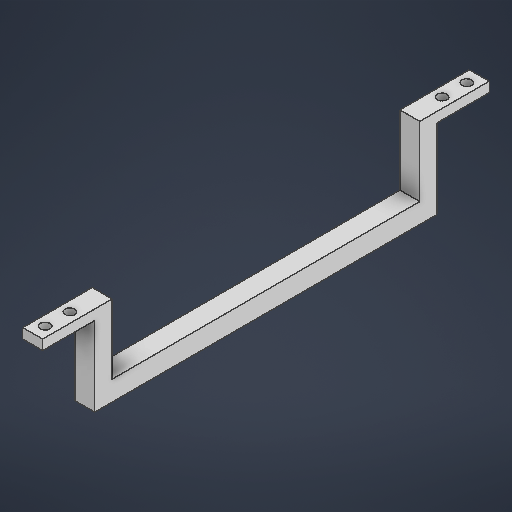
# Autodesk Inventor part: side_wall2
Saved by Autodesk Inventor 2026.1 (Build 301233000, 233)
## iProperties
Created: 2026-03-22
Part Number: side_wall2
Material: Generic
Document SubType Name: Modeling
Designer: emanuel
Density: 1 g/cm^3
Appearance: Default
Author: emanuel
Autodesk Inventor part; units mm, degrees
ref_plane "YZ Plane" through (0, 0, 0) normal (1, 0, 0) x (0, 1, 0)
ref_plane "XZ Plane" through (0, 0, 0) normal (0, 1, 0) x (-1, 0, 0)
ref_plane "XY Plane" through (0, 0, 0) normal (0, 0, 1) x (1, 0, 0)
sketch "Sketch1" plane through (0, 0, 0) normal (0, 1, 0) x (-1, 0, 0)
  circle A0 centre (0, 0) radius 2
  line L0 (0, 0) -> (0, -10)
  circle A1 centre (0, -10) radius 2
  line L1 (0, 0) -> (4, 0)
  line L2 (4, 0) -> (4, 5)
  line L3 (4, 5) -> (0, 5)
  line L4 (0, 5) -> (0, 0)
  line L5 (0, -10) -> (-4, -10)
  line L6 (-4, -10) -> (-4, -15)
  line L7 (-4, -15) -> (0, -15)
  line L8 (0, -15) -> (0, -10)
  line L9 (4, 5) -> (-4, 5)
  line L10 (-4, 5) -> (-4, -15)
  line L11 (-4, -15) -> (4, -15)
  line L12 (4, -15) -> (4, 5)
  line L13 (4, -15) -> (-4, -15)
  line L14 (-4, -15) -> (-4, -23)
  line L15 (-4, -23) -> (4, -23)
  line L16 (4, -23) -> (4, -15)
  line L17 (0, -10) -> (0, -85)
  line L18 (0, -85) -> (10, -85)
  circle A2 centre (0, -170) radius 2
  line L19 (0, -170) -> (0, -160)
  circle A3 centre (0, -160) radius 2
  line L20 (0, -170) -> (4, -170)
  line L21 (4, -170) -> (4, -175)
  line L22 (4, -175) -> (0, -175)
  line L23 (0, -175) -> (0, -170)
  line L24 (0, -160) -> (-4, -160)
  line L25 (-4, -160) -> (-4, -155)
  line L26 (-4, -155) -> (0, -155)
  line L27 (0, -155) -> (0, -160)
  line L28 (4, -175) -> (-4, -175)
  line L29 (-4, -175) -> (-4, -155)
  line L30 (-4, -155) -> (4, -155)
  line L31 (4, -155) -> (4, -175)
  line L32 (4, -155) -> (-4, -155)
  line L33 (-4, -155) -> (-4, -147)
  line L34 (-4, -147) -> (4, -147)
  line L35 (4, -147) -> (4, -155)
  dimension "d0" = 4
  dimension "d1" = 10
  dimension "d2" = 4
  dimension "d3" = 4
  dimension "d4" = 5
  dimension "d5" = 4
  dimension "d6" = 5
  dimension "d7" = 8
  dimension "d8" = 75
  dimension "d9" = 10
  constraints: 72 end point, 15 symmetric about line, 8 parallel, 5 perpendicular, 4 centre point, 4 coincident, 4 horizontal, 3 point on line, 1 vertical, 2 other
  measures "d0" diameter of A0
  measures "d1" distance of L0.start L0.end
  measures "d2" diameter of A1
  measures "d3" distance of L3.end L2.end
  measures "d4" distance of L2.end L1.end
  measures "d5" distance of L7.end L6.end
  measures "d6" distance of L6.end L5.end
  measures "d7" distance of L14.end L13.end
  measures "d8" distance of L5.start L17.end
  measures "d9" distance of L17.end L18.end
extrude "Extrusion1" add sketch "Sketch1" along normal blind 4 contours L1 L12 L11 L8 A1 L0 A0 | A0 L4 L3 L2 L1 | A0 L0 A1 L5 L10 L9 L4 | L16 L15 L17 L11 | A1 L8 L7 L6 L5 | L17 L15 L14 L7 | L20 L21 L22 L23 A2 | A2 L19 A3 L27 L30 L31 L20 | A2 L23 L28 L29 L24 A3 L19 | L30 L26 L33 L34 L35 | L24 L25 L26 L27 A3
sketch "Sketch2" plane through (0, 0, 0) normal (0, -1, 0) x (1, 0, 0)
  line L0 (4, -23) -> (-4, -23) projected
  line L1 (4, 5) -> (4, -23) projected
  line L2 (-4, -23) -> (4, -23)
  line L3 (4, -23) -> (4, -16)
  line L4 (4, -16) -> (-4, -16)
  line L5 (-4, -16) -> (-4, -23)
  line L6 (-4, -147) -> (4, -147) projected
  line L7 (-4, -147) -> (4, -147)
  line L8 (4, -147) -> (4, -154)
  line L9 (4, -154) -> (-4, -154)
  line L10 (-4, -154) -> (-4, -147)
  point P0 (0, 0)
  dimension "d12" = 7
  dimension "d13" = 7
  constraints: 16 end point, 4 parallel, 2 horizontal, 2 perpendicular, 2 point on line
  measures "d12" distance of L3.end L2.end
  measures "d13" distance of L7.end L8.end
extrude "Extrusion2" add sketch "Sketch2" along normal blind 32
sketch "Sketch3" plane through (0, -32, 0) normal (0, -1, 0) x (1, 0, 0)
  line L0 (4, -154) -> (4, -147) projected
  line L1 (-4, -16) -> (-4, -23) projected
  line L2 (4, -154) -> (-4, -154)
  line L3 (-4, -154) -> (-4, -16)
  line L4 (-4, -16) -> (4, -16)
  line L5 (4, -16) -> (4, -154)
  point P0 (0, 0)
  constraints: 8 end point, 2 parallel, 1 horizontal, 1 perpendicular
extrude "Extrusion3" add sketch "Sketch3" against normal blind 8
body "Solid1"
